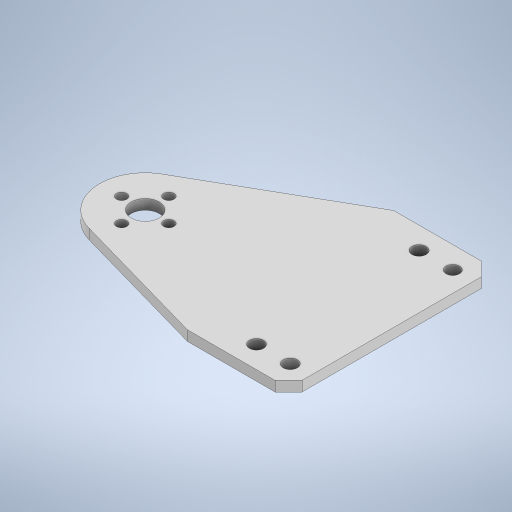
# Autodesk Inventor part: sh1-short
Saved by Autodesk Inventor 2024 (Build 280153000, 153)
## iProperties
Created: 2023-08-14
Part Number: sh1-short
Material: 常规
Document SubType Name: Modeling
Designer: wya
Density: 1 g/cm^3
Appearance: 默认
Author: wya
Autodesk Inventor part; units mm, degrees
ref_plane "YZ Plane" through (0, 0, 0) normal (1, 0, 0) x (0, 1, 0)
ref_plane "XZ Plane" through (0, 0, 0) normal (0, 1, 0) x (-1, 0, 0)
ref_plane "XY Plane" through (0, 0, 0) normal (0, 0, 1) x (1, 0, 0)
sketch "草图1" plane through (0, 0, 0) normal (0, 1, 0) x (-1, 0, 0)
  line L0 (37, 0) -> (0, 0)
  line L1 (0, 0) -> (0, -27)
  line L2 (0, -27) -> (37, -27)
  line L3 (37, -27) -> (37, 0)
  circle A0 centre (37, -13.5) radius 13.5
  line L4 (0, 0) -> (-30, 0)
  line L5 (-30, 0) -> (-30, -50.2)
  line L6 (-30, -50.2) -> (0, -50.2)
  line L7 (0, -50.2) -> (0, 0)
  line L8 (0, 11) -> (-30, 11)
  line L9 (-30, 11) -> (-30, 0)
  line L10 (-30, 0) -> (0, 0)
  line L11 (0, 0) -> (0, 11)
  line L12 (0, -13.5) -> (-5.5, -13.5)
  circle A1 centre (-24, 4.5) radius 2.1
  circle A2 centre (-14, 4.5) radius 2.1
  line L13 (-14, 4.5) -> (-24, 4.5)
  line L14 (-14, 4.5) -> (-24, 4.5)
  line L15 (-24, 4.5) -> (-24, -43.7)
  line L16 (-24, -43.7) -> (-14, -43.7)
  line L17 (-14, -43.7) -> (-14, 4.5)
  circle A3 centre (-14, -43.7) radius 2.1
  circle A4 centre (-24, -43.7) radius 2
  line L18 (0, 11) -> (40.6758, -0.5101)
  line L19 (43.6996, -25.2203) -> (0, -50.2)
  circle A5 centre (37, -13.5) radius 4.15
  circle A6 centre (37, -20.5) radius 1.525
  circle A7 centre (37, -6.5) radius 1.525
  circle A8 centre (44, -13.5) radius 1.525
  circle A9 centre (30, -13.5) radius 1.525
  circle A10 centre (37, -13.5) radius 7
  line L20 (37, -13.5) -> (63.1942, -13.5)
  point P0 (0, -13.5)
  dimension "d0" = 27
  dimension "d1" = 37
  dimension "d2" = 30
  dimension "d3" = 24
  dimension "d4" = 4.2
  dimension "d5" = 10
  dimension "d6" = 18
  dimension "d7" = 11
  dimension "d8" = 48.2
  dimension "d9" = 4.2
  dimension "d10" = 4
  dimension "d11" = 6.5
  dimension "d12" = 8.3
  dimension "d13" = 14
  dimension "d14" = 3.05
  constraints: 43 end point, 11 centre point, 9 parallel, 8 point on line, 7 point on circle, 5 horizontal, 5 perpendicular, 4 coincident, 4 equal radius, 2 collinear, 2 midpoint, 2 tangent
  measures "d0" distance of L2.end L0.start
  measures "d1" distance between parallel lines of L1 L3
  measures "d2" distance between parallel lines of L5 L1
  measures "d3" distance from line of L1 L13.end
  measures "d4" diameter of A2
  measures "d5" distance of L13.start L13.end
  measures "d6" distance between parallel lines of L12 L13
  measures "d7" distance between parallel lines of L4 L8
  measures "d8" distance between parallel lines of L16 L13
  measures "d9" diameter of A3
  measures "d10" diameter of A4
  measures "d11" distance between parallel lines of L6 L16
  measures "d12" diameter of A5
  measures "d13" diameter of A10
  measures "d14" diameter of A7
extrude "拉伸1" add sketch "草图1" along normal blind 3 contours A0 L2 L1 L0 | A0 L20 A8 A10 A7 L3 | L0 L11 L18 A0 | L3 A7 A10 A9 A6 A0 | L1 L7 L6 L5 L4 L15 A4 L16 A3 L17 | L4 L17 A2 L13 A1 L15 L9 L8 L11 | A0 L19 L7 L2 | L3 A6 A10 A8 L20 A0 | L17 A3 L16 A4 L15 L4 | L4 L15 A1 L13 A2 L17 | A7 L3 A5 A6 A10 A9 | A7 A10 A8 L20 A5 L3 | A10 A6 L3 A5 L20 A8
chamfer "倒角1" distance 4 angle 45 2 edges at (30, 1.5, -50.2) (30, 1.5, 11)
